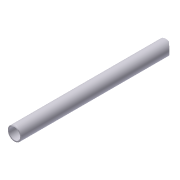
# Autodesk Inventor part: FE-00006-10
Saved by Autodesk Inventor 2012 (Build 160160000, 160)
## iProperties
Created: 2008-05-25
Part Number: FE-00006-10
Document SubType Name: Modeling
Designer: firstuser
Density: 1 g/cm^3
Mass: 200.109 g
Surface Area: 1130.46 cm^2
Volume: 200.109 cm^3
Material: Default
Author: firstuser
Autodesk Inventor part; units mm, degrees
ref_plane "XZ Plane" through (0, 0, 0) normal (0, 1, 0) x (-1, 0, 0)
ref_plane "XY Plane" through (0, 0, 0) normal (0, 0, 1) x (1, 0, 0)
sketch "Sketch1" plane through (0, 0, 0) normal (0, 0, 1) x (1, 0, 0)
  circle A0 centre (0, 0) radius 21.0312
  circle A1 centre (0, 0) radius 17.4625
  dimension "d0" = 34.925
  dimension "d1" = 42.0624
  constraints: 2 centre point, 1 coincident
  measures "d0" diameter of A1
  measures "d1" diameter of A0
extrude "Extrusion1" add sketch "Sketch1" along normal blind 469.1126
ref_plane "Work Plane1" through (0, 0, 0) normal (1, 0, 0) x (0, 0, 1)
sketch "Sketch2" plane through (0, 0, 0) normal (1, 0, 0) x (0, 0, 1)
  circle A0 centre (-11.0998, 0) radius 21.4312
  line L0 (-132.8598, 0) -> (569.4413, 0) projected
  line L1 (469.1126, 17.4625) -> (469.1126, -17.4625) projected
  dimension "d5" = 42.8625
  dimension "d6" = 480.2124
  constraints: 1 centre point, 1 point on line
  measures "d5" diameter of A0
  measures "d6" distance from line of L1 A0.centre
extrude "Extrusion2" cut sketch "Sketch2" against normal mid plane 1066.8
sketch "Sketch3" plane through (0, 0, 0) normal (1, 0, 0) x (0, 0, 1)
  line L0 (0, -21.0312) -> (469.1126, -21.0312) projected
  line L1 (469.1126, 17.4625) -> (469.1126, -17.4625) projected
  line L2 (469.1126, 21.0312) -> (469.1126, -21.0312) projected
  line L3 (483.7746, -29.5638) -> (456.7933, -29.5638)
  line L4 (456.7933, -29.5638) -> (456.7933, -21.0312)
  line L5 (456.7933, -21.0312) -> (462.7626, -21.0312)
  line L6 (469.1126, -14.6812) -> (469.1126, -8.6172)
  line L7 (469.1126, -8.6172) -> (483.7746, -8.6172)
  line L8 (483.7746, -8.6172) -> (483.7746, -29.5638)
  arc A0 (462.7626, -21.0312) -> (469.1126, -14.6812) centre (462.7626, -14.6812) ccw
  dimension "d9" = 6.35
  constraints: 12 end point, 4 parallel, 2 collinear, 2 perpendicular, 2 point on circle, 2 tangent, 1 centre point
  measures "d9" radius of A0
extrude "Extrusion3" cut sketch "Sketch3" against normal mid plane 1066.8
body "Solid1"
